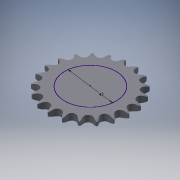
# Autodesk Inventor part: BigSprocket11
Saved by Autodesk Inventor 2016 (Build 200138000, 138)
## iProperties
Created: 2016-05-10
Part Number: BigSprocket11
Material: Steel
Document SubType Name: Modeling
Designer: hesaon
Density: 1 g/cm^3
Appearance: Steel
CustomPartVersion: 1
Author: hesaon
Autodesk Inventor part; units mm, degrees
ref_plane "YZ Plane" through (0, 0, 0) normal (1, 0, 0) x (0, 1, 0)
ref_plane "XZ Plane" through (0, 0, 0) normal (0, 1, 0) x (-1, 0, 0)
sketch "Theoretical Tooth Profile" plane through (0, 0, 0) normal (0, 0, 1) x (1, 0, 0)
  circle A0 centre (0, 0) radius 31.954 construction
  line L0 (0, 0) -> (0, 31.954) construction
  line L1 (0, 0) -> (9.4186, 30.5344) construction
  circle A1 centre (0, 0) radius 34.4546
  arc A2 (-2.5319, 29.9861) -> (2.5319, 29.9861) centre (0, 31.954) ccw
  line L2 (0, 31.954) -> (9.4186, 30.5344) construction
  line L3 (0, 31.954) -> (4.0109, 35.0716) construction
  line L4 (4.0109, 35.0716) -> (-3.6438, 31.8972) construction
  arc A3 (4.8724, 34.1084) -> (3.9503, 32.6364) centre (8.7907, 30.629) ccw
  arc A4 (-3.9503, 32.6364) -> (-4.8724, 34.1084) centre (-8.7907, 30.629) ccw
  line L5 (-8.7907, 30.629) -> (-3.9503, 32.6364) construction
  arc A5 (-3.6438, 31.8972) -> (-2.5319, 29.9861) centre (4.0109, 35.0716) ccw
  line L6 (-3.6438, 31.8972) -> (-3.9503, 32.6364)
  arc A6 (2.5319, 29.9861) -> (3.6438, 31.8972) centre (-4.0109, 35.0716) ccw
  line L7 (3.9503, 32.6364) -> (3.6438, 31.8972)
  line L8 (0, 0) -> (5.1352, 34.0698) construction
  point P0 (4.7093, 31.2442)
  dimension "d0" = 63.9081
  dimension "d2" = 17.143
  dimension "d3" = 3.2067
  dimension "d10" = 127.857
  dimension "d11" = 15.333
  dimension "d12" = 5.08
  dimension "d13" = 8.2867
  dimension "d14" = 8.89
  dimension "d23" = 2.8575
  constraints: 18 end point, 15 point on circle, 7 centre point, 3 coincident, 3 point on line, 3 symmetric about line, 3 tangent, 1 equal radius, 1 midpoint, 1 parallel, 1 vertical, 1 other
  measures "d0" diameter of A0
  measures "d2" angle of L1 L0
  measures "d3" radius of A2
  measures "d10" angle of L3 L0
  measures "d11" angle of L4 L3
  measures "d12" distance of L2.start L3.end
  measures "d13" distance of L3.end L4.end
  measures "d14" distance of A3.centre L0.end
  measures "d23" distance from line of L8.end L2
sketch "Tooth Profile" plane through (0, 0, 0) normal (0, 0, 1) x (1, 0, 0)
  arc A0 (-2.9702, 30.7453) -> (2.9702, 30.7453) centre (0, 31.954) ccw
  arc A1 (4.7964, 34.1191) -> (2.9702, 30.7453) centre (19.2036, 24.1395) ccw
  arc A2 (-2.9702, 30.7453) -> (-4.7964, 34.1191) centre (-19.2036, 24.1395) ccw
  line L0 (0, 0) -> (0, 31.954) construction
  line L1 (0, 31.954) -> (2.9702, 30.7453) construction
  line L2 (0, 31.954) -> (-2.9702, 30.7453) construction
  circle A3 centre (0, 0) radius 34.4546 projected
  dimension "d44" = 135.714
  dimension "d45" = 17.526
  dimension "d46" = 3.2067
  constraints: 9 point on circle, 6 end point, 3 centre point, 2 tangent, 1 coincident, 1 equal radius, 1 vertical, 1 other
  measures "d44" angle of L2 L1
  measures "d45" radius of A1
  measures "d46" radius of A0
sketch "Section Profile" plane through (0, 0, 0) normal (1, 0, 0) x (0, 1, 0)
  line L0 (34.4546, 0) -> (-34.4546, 0) projected
  line L1 (23.1209, 2.6598) -> (-23.1209, 2.6598)
  line L2 (-23.1209, 2.6598) -> (-23.1209, -2.6598)
  line L3 (-23.1209, -2.6598) -> (23.1209, -2.6598)
  line L4 (23.1209, -2.6598) -> (23.1209, 2.6598)
  line L5 (23.1209, 2.6598) -> (34.4546, 2.6598) construction
  line L6 (34.4546, 2.6598) -> (34.4546, -2.6598) construction
  line L7 (34.4546, -2.6598) -> (23.1209, -2.6598) construction
  line L8 (23.1209, -2.6598) -> (23.1209, 2.6598)
  arc A0 (34.4546, 1.4692) -> (29.8434, 2.6598) centre (29.8434, -6.8652) ccw
  arc A1 (29.8434, -2.6598) -> (34.4546, -1.4692) centre (29.8434, 6.8652) ccw
  line L9 (29.8434, 2.6598) -> (0, 2.6598)
  line L10 (0, 2.6598) -> (0, -2.6598)
  line L11 (0, -2.6598) -> (29.8434, -2.6598)
  line L12 (0, 2.6598) -> (0, -2.6598)
  line L13 (34.4546, 1.4692) -> (34.4546, -1.4692)
  point P0 (0, 0)
  point P1 (0, 0)
  dimension "d30" = 5.3196
  dimension "d31" = 46.2418
  dimension "d32" = 5.3196
  dimension "d33" = 1.1906
  dimension "d34" = 9.525
  dimension "d43" = 2.6598
  constraints: 26 end point, 7 midpoint, 5 perpendicular, 4 parallel, 4 point on circle, 3 point on line, 3 symmetric about line, 2 centre point, 2 horizontal, 2 tangent, 1 collinear, 1 other
  measures "d30" distance between parallel lines of L7 L5
  measures "d31" distance between parallel lines of L2 L4
  measures "d32" distance between parallel lines of L3 L1
  measures "d33" distance from line of L13.start L5
  measures "d34" radius of A0
  measures "d43" distance between parallel lines of L3 L0
revolve "Shroud" add sketch "Section Profile" angle 360 about axis through (0, 0, 2.6598) along (0, 0, -1) contours L10 L3 L2 L0 | L0 L2 L1 L10
revolve "Strand" add sketch "Section Profile" angle 360 about axis through (0, 0, 2.6598) along (0, 0, -1) contours L13 A1 L11 L4 L0 | L0 L4 L9 A0 L13 | L4 L3 L10 L0 | L0 L10 L1 L4
pattern_of_one "Strand Pattern"
extrude "Theoretical Tooth" cut sketch "Theoretical Tooth Profile" along normal through all both and the other way through all contours A3 L7 A6 A2 A5 L6 A4 A1 picked at (0, 32.5265)
extrude "Tooth" [suppressed]
pattern_circular "Tooth Pattern" count 21 over 360 about axis through (0, 0, -10) along (0, 0, 1) of "Theoretical Tooth"
ref_plane "Timing Plane" through (0, 31.954, 0) normal (1, 0, 0) x (0, 1, 0)
sketch "Sketch4" plane through (0, 31.954, 2.6598) normal (0, 0, 1) x (1, 0, 0)
  circle A0 centre (0, -31.954) radius 21
  dimension "d51" = 42
  constraints: 1 centre point, 1 coincident
  measures "d51" diameter of A0
equation "\"d3\" = 0.5 * da_Dr + da_SC"
equation "\"d12\" = 0.8 * da_Dr"
equation "\"d13\" = 1.3 * da_Dr + da_SC"
equation "\"d14\" = 1.4 * da_Dr"
equation "\"d23\" = da_Ha"
equation "\"d44\" = da_Alfa"
equation "\"d45\" = da_Re"
equation "\"d46\" = da_Ri"
equation "\"d30\" = da_Bf"
equation "\"d31\" = da_Ds"
equation "\"d32\" = da_Bs"
equation "\"d33\" = da_Ba"
equation "\"d34\" = da_Rx"
equation "\"d40\" = da_pt"
equation "\"form_type\" = 0"
equation "\"da_p\" = 9.525"
equation "\"da_Dr\" = 6.35"
equation "\"da_SC\" = 0.03175"
equation "\"da_Ha\" = 2.8575"
equation "\"da_pt\" = 10.24"
equation "\"da_Bf\" = 5.3196"
equation "\"da_Ba\" = 1.19063"
equation "\"da_Rx\" = 9.525"
equation "\"da_Ra\" = 0.381"
equation "\"da_Bs\" = 5.3196"
equation "\"da_Ds\" = 46.24185"
equation "\"da_Re\" = 17.526"
equation "\"da_Ri\" = 3.20675"
equation "\"da_Alfa\" = 135.714deg"
body "Solid1"
